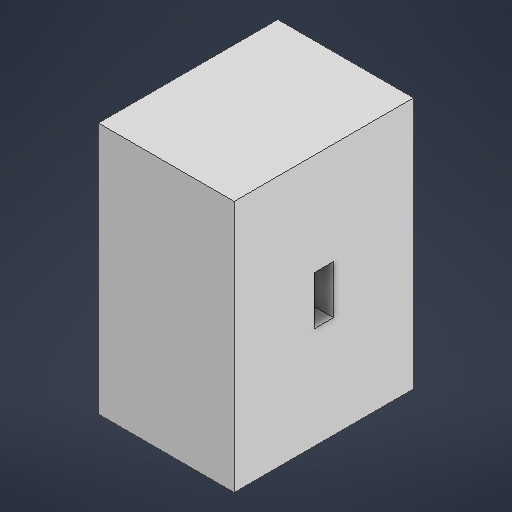
# Autodesk Inventor part: Magnet
Saved by Autodesk Inventor 2026.2 (Build 302298010, 298A)
## iProperties
Created: 2026-09-21
Part Number: Magnet
Material: Generic
Document SubType Name: Modeling
Designer: aiden
Density: 1 g/cm^3
Appearance: Default
Author: aiden
Autodesk Inventor part; units mm, degrees
ref_plane "YZ Plane" through (0, 0, 0) normal (1, 0, 0) x (0, 1, 0)
ref_plane "XZ Plane" through (0, 0, 0) normal (0, 1, 0) x (-1, 0, 0)
ref_plane "XY Plane" through (0, 0, 0) normal (0, 0, 1) x (1, 0, 0)
sketch "Sketch1" plane through (0, 0, 0) normal (0, 1, 0) x (-1, 0, 0)
  line L0 (-44.45, -58.7375) -> (44.45, -58.7375)
  line L1 (44.45, -58.7375) -> (44.45, 58.7375)
  line L2 (44.45, 58.7375) -> (-44.45, 58.7375)
  line L3 (-44.45, 58.7375) -> (-44.45, -58.7375)
  line L4 (-44.45, -58.7375) -> (44.45, 58.7375) construction
  line L5 (44.45, -58.7375) -> (-44.45, 58.7375) construction
  point P0 (0, 0)
  dimension "d0" = 88.9
  dimension "d1" = 117.475
  constraints: 12 end point, 2 midpoint, 2 parallel, 1 horizontal, 1 perpendicular
  measures "d0" distance of L2.end L1.end
  measures "d1" distance of L1.end L0.end
extrude "Extrusion1" add sketch "Sketch1" along normal blind 165.1
sketch "Sketch2" plane through (44.45, 0, 58.7375) normal (1, 0, 0) x (0, 0, -1)
  line L0 (58.7375, 0) -> (58.7375, 165.1) construction
  line L1 (117.475, 165.1) -> (0, 165.1) construction
  line L2 (65.0875, 66.675) -> (52.3875, 66.675) construction
  line L3 (52.3875, 66.675) -> (52.3875, 98.425) construction
  line L4 (52.3875, 98.425) -> (65.0875, 98.425) construction
  line L5 (65.0875, 98.425) -> (65.0875, 66.675) construction
  line L6 (65.0875, 66.675) -> (52.3875, 98.425) construction
  line L7 (52.3875, 66.675) -> (65.0875, 98.425) construction
  line L8 (52.3875, 98.425) -> (65.0875, 98.425)
  line L9 (65.0875, 66.675) -> (65.0875, 98.425)
  line L10 (65.0875, 66.675) -> (52.3875, 66.675)
  line L11 (52.3875, 98.425) -> (52.3875, 66.675)
  point P0 (58.7375, 82.55)
  dimension "d4" = 12.7
  dimension "d5" = 31.75
  constraints: 22 end point, 5 equal length, 4 midpoint, 2 horizontal, 1 perpendicular
  measures "d4" distance of L3.end L4.end
  measures "d5" distance of L2.end L3.end
extrude "Extrusion2" cut sketch "Sketch2" against normal blind 165.1
body "Solid1"
